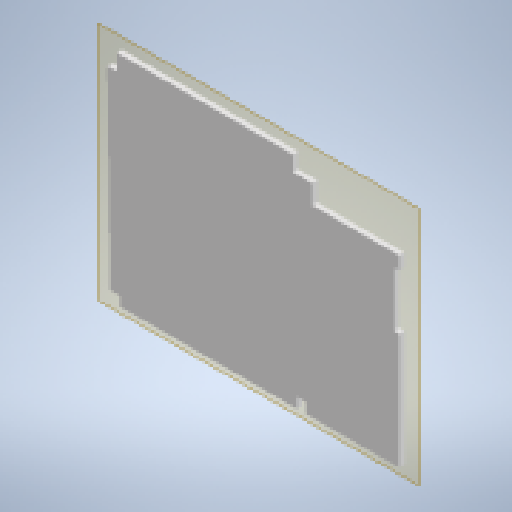
# Autodesk Inventor part: Suelo
Saved by Autodesk Inventor 2024 (Build 280153000, 153)
## iProperties
Created: 2024-04-05
Part Number: Suelo
Material: Genérico
Document SubType Name: Modeling
Designer: sergi
Density: 1 g/cm^3
Appearance: Valor por defecto
Author: sergi
Autodesk Inventor part; units mm, degrees
ref_plane "YZ Plane" through (0, 0, 0) normal (1, 0, 0) x (0, 1, 0)
ref_plane "XZ Plane" through (0, 0, 0) normal (0, 1, 0) x (-1, 0, 0)
ref_plane "XY Plane" through (0, 0, 0) normal (0, 0, 1) x (1, 0, 0)
ref_plane "Plano de trabajo1" through (0, 0, 0) normal (0, 0, 1) x (1, 0, 0)
sketch "Boceto1" plane through (0, 0, 0) normal (0, 0, 1) x (1, 0, 0)
  line L0 (2750.7331, 132.5) -> (2750.7331, -2057.5) projected
  line L1 (2650.7331, 132.5) -> (2750.7331, 132.5) projected
  line L2 (2650.7331, -1957.5) -> (2650.7331, 132.5) projected
  line L3 (1090.7331, -1957.5) -> (2650.7331, -1957.5) projected
  line L4 (1090.7331, -1762.5) -> (1090.7331, -1957.5) projected
  line L5 (715.7331, -1762.5) -> (1090.7331, -1762.5) projected
  line L6 (715.7331, -1957.5) -> (715.7331, -1762.5) projected
  line L7 (-2414.2669, -1957.5) -> (715.7331, -1957.5) projected
  line L8 (-2414.2669, -1782.5) -> (-2414.2669, -1957.5) projected
  line L9 (-2599.2669, -1782.5) -> (-2414.2669, -1782.5) projected
  line L10 (-2649.2669, 1652.5) -> (-2599.2669, -1782.5) projected
  line L11 (-2469.2669, 1652.5) -> (-2649.2669, 1652.5) projected
  line L12 (-2469.2669, 1957.5) -> (-2469.2669, 1652.5) projected
  line L13 (640.7331, 1957.5) -> (-2469.2669, 1957.5) projected
  line L14 (640.7331, 1667.5) -> (640.7331, 1957.5) projected
  line L15 (1005.7331, 1667.5) -> (640.7331, 1667.5) projected
  line L16 (1005.7331, 1307.5) -> (1005.7331, 1667.5) projected
  line L17 (2650.7331, 1307.5) -> (1005.7331, 1307.5) projected
  line L18 (2650.7331, 1162.5) -> (2650.7331, 1307.5) projected
  line L19 (2750.7331, 1162.5) -> (2650.7331, 1162.5) projected
  line L20 (2750.7331, 1407.5) -> (2750.7331, 1162.5) projected
  line L21 (1105.7331, 1407.5) -> (2750.7331, 1407.5) projected
  line L22 (1105.7331, 1767.5) -> (1105.7331, 1407.5) projected
  line L23 (740.7331, 1767.5) -> (1105.7331, 1767.5) projected
  line L24 (740.7331, 2057.5) -> (740.7331, 1767.5) projected
  line L25 (-2569.2669, 2057.5) -> (740.7331, 2057.5) projected
  line L26 (-2569.2669, 1752.5) -> (-2569.2669, 2057.5) projected
  line L27 (-2750.7331, 1752.5) -> (-2569.2669, 1752.5) projected
  line L28 (-2697.8219, -1882.5) -> (-2750.7331, 1752.5) projected
  line L29 (-2514.2669, -1882.5) -> (-2697.8219, -1882.5) projected
  line L30 (-2514.2669, -2057.5) -> (-2514.2669, -1882.5) projected
  line L31 (2650.7331, 1162.5) -> (2750.7331, 1162.5) projected
  line L32 (2650.7331, 132.5) -> (2650.7331, 1162.5) projected
  line L33 (2750.7331, 132.5) -> (2650.7331, 132.5) projected
  line L34 (2750.7331, 132.5) -> (2750.7331, 1162.5) projected
  line L35 (2650.7331, 1162.5) -> (2750.7331, 1162.5) projected
  line L36 (2650.7331, 132.5) -> (2650.7331, 1162.5) projected
  line L37 (2750.7331, 132.5) -> (2650.7331, 132.5) projected
  line L38 (2750.7331, 132.5) -> (2750.7331, 1162.5) projected
  line L39 (2750.7331, -2057.5) -> (-2514.2669, -2057.5) projected
  point P0 (0, 0)
  point P1 (990.7331, -2057.5)
  point P2 (815.7331, -2057.5)
extrude "Extrusión1" add sketch "Boceto1" along normal blind 100
sketch "Boceto2" plane through (0, 0, 0) normal (0, 0, -1) x (-1, 0, 0)
  line L0 (-1930.7331, 1162.5) -> (-2650.7331, 1162.5)
  arc A0 (-2650.7331, 442.5) -> (-1930.7331, 1162.5) centre (-2650.7331, 1162.5) ccw
  arc A1 (-2340.7331, 132.5) -> (-2650.7331, 442.5) centre (-2650.7331, 132.5) ccw
  line L1 (-2650.7331, 132.5) -> (-2340.7331, 132.5)
  point P0 (0, 0)
  constraints: 4 end point, 4 point on circle, 2 centre point, 1 coincident
